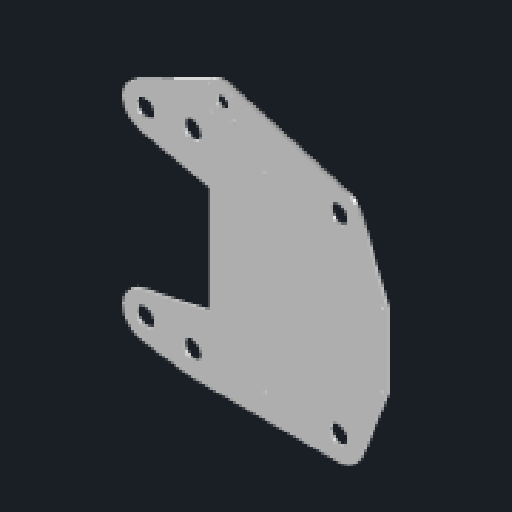
# Autodesk Inventor part: OUTK_002_ShotPlateNoReceptacle
Saved by Autodesk Inventor 2024.2 (Build 282272000, 272)
## iProperties
Created: 2024-11-24
Part Number: OUTK_002_ShotPlateNoReceptacle
Material: Aluminum 6061
Document SubType Name: Modeling
Designer: Bryan
Density: 2.7 g/cm^3
Appearance: Aluminum - Flat
Mass: 844.378 g
Surface Area: 1588.21 cm^2
Volume: 312.733 cm^3
Author: Bryan
Autodesk Inventor part; units mm, degrees
ref_plane "YZ Plane" through (0, 0, 0) normal (1, 0, 0) x (0, 1, 0)
ref_plane "XZ Plane" through (0, 0, 0) normal (0, 1, 0) x (-1, 0, 0)
ref_plane "XY Plane" through (0, 0, 0) normal (0, 0, 1) x (1, 0, 0)
sketch "Sketch1" plane through (0, 0, 0) normal (0, 0, 1) x (1, 0, 0)
  circle A0 centre (239.2032, 0) radius 130.175 projected
  arc A1 (74.585, 187.96) -> (69.5611, 187.6187) centre (74.585, 150.8125) ccw projected
  line L0 (69.5611, 187.6187) -> (-4.7233, 177.4791) projected
  arc A2 (-4.7233, 177.4791) -> (-7.5024, 108.7653) centre (0, 142.875) ccw projected
  line L1 (-7.5024, 108.7653) -> (102.6782, 84.5312) projected
  line L2 (102.6782, 84.5312) -> (102.6782, -84.5312) projected
  line L3 (102.6782, -84.5312) -> (-7.5024, -108.7653) projected
  arc A3 (-7.5024, -108.7653) -> (-5.1627, -177.4163) centre (0, -142.875) ccw projected
  line L4 (-5.1627, -177.4163) -> (68.953, -188.4939) projected
  arc A4 (68.953, -188.4939) -> (74.585, -188.9125) centre (74.585, -150.8125) ccw projected
  line L5 (74.585, -188.9125) -> (305.8782, -188.9125) projected
  arc A5 (305.8782, -188.9125) -> (341.4207, -164.5364) centre (305.8782, -150.8125) ccw projected
  line L6 (341.4207, -164.5364) -> (381.652, -60.3445) projected
  arc A6 (381.652, -60.3445) -> (382.0782, -58.0572) centre (375.7282, -58.0572) ccw projected
  line L7 (382.0782, -58.0572) -> (382.0782, 58.0572) projected
  arc A7 (382.0782, 58.0572) -> (381.6323, 60.3949) centre (375.7282, 58.0572) ccw projected
  line L8 (381.6323, 60.3949) -> (340.4169, 164.488) projected
  arc A8 (340.4169, 164.488) -> (305.8782, 187.96) centre (305.8782, 150.8125) ccw projected
  circle A9 centre (74.585, -150.8125) radius 14.2875 projected
  circle A10 centre (74.585, 150.8125) radius 14.2875 projected
  circle A11 centre (190.2316, 150.8125) radius 3.2512 projected
  circle A12 centre (190.2316, -150.8125) radius 3.2512 projected
  circle A13 centre (375.7282, -58.0572) radius 3.2512 projected
  circle A14 centre (375.7282, 58.0572) radius 3.2512 projected
  circle A15 centre (305.8782, 150.8125) radius 14.2875 projected
  circle A16 centre (305.8782, -150.8125) radius 14.2875 projected
  circle A17 centre (0, -142.875) radius 14.2875 projected
  circle A18 centre (0, 142.875) radius 14.2875 projected
  circle A19 centre (112.9698, 216.6384) radius 38.1 construction
  circle A20 centre (112.9698, 216.6384) radius 19.1008 construction
  circle A21 centre (112.9698, 216.6384) radius 9.6202
  circle A22 centre (133.1724, 201.2431) radius 2.4892
  circle A23 centre (128.3651, 236.841) radius 2.4892
  circle A24 centre (92.7672, 232.0337) radius 2.4892
  circle A25 centre (97.5746, 196.4358) radius 2.4892
  line L9 (84.856, 243.5486) -> (92.7672, 232.0337) construction
  line L10 (128.3651, 236.841) -> (132.9386, 250.0419) construction
  circle A26 centre (112.9698, 216.6384) radius 25.4 construction
  line L11 (112.9698, 216.6384) -> (305.8782, -150.8125) construction
  circle A27 centre (74.585, 150.8125) radius 38.1 construction
  line L12 (318.039, 185.9131) -> (125.4424, 252.639)
  line L13 (91.3948, 248.041) -> (-19.7772, 171.6608)
  arc A28 (125.4424, 252.639) -> (91.3948, 248.041) centre (112.9698, 216.6384) ccw
  dimension "d192" = 50.8
  dimension "d186" = 76.2
  dimension "d187" = 38.2016
  dimension "d188" = 19.2405
  dimension "d189" = 4.9784
  dimension "d190" = 360
  dimension "d193" = 415.0106
  constraints: 10 end point, 9 centre point, 6 coincident, 6 point on circle, 5 tangent, 2 perpendicular, 2 point on line, 1 concentric, 1 equal length, 1 equal radius, 12 other
  measures "d186" diameter of A19
  measures "d187" diameter of A20
  measures "d188" diameter of A21
  measures "d189" diameter of A22
  measures "d193" distance of L11.start L11.end
extrude "Extrusion1" add sketch "Sketch1" along normal mid plane 4.7625 contours A0 | L13 A28 L12 A8 L8 A7 L7 A6 L6 A5 L5 A4 L4 A3 L3 L2 L1 A2
sketch "Sketch2" plane through (0, 0, -2.3813) normal (0, 0, -1) x (-1, 0, 0)
  line L0 (7.573, -108.7809) -> (-101.6, -84.5312) projected
  line L1 (-101.6, -84.5312) -> (-101.6, 84.5312) projected
  line L2 (-101.6, 84.5312) -> (7.573, 108.7809) projected
  arc A0 (7.573, 108.7809) -> (16.0837, 173.8761) centre (0, 142.875) ccw projected
  arc A1 (-315.0883, 186.5069) -> (-339.3386, 164.488) centre (-304.8, 150.8125) ccw projected
  line L3 (-339.3386, 164.488) -> (-380.554, 60.3949) projected
  arc A2 (-380.554, 60.3949) -> (-381, 58.0572) centre (-374.65, 58.0572) ccw projected
  line L4 (-381, 58.0572) -> (-381, -58.0572) projected
  arc A3 (-381, -58.0572) -> (-380.5737, -60.3445) centre (-374.65, -58.0572) ccw projected
  line L5 (-380.5737, -60.3445) -> (-340.3424, -164.5364) projected
  arc A4 (-340.3424, -164.5364) -> (-304.8, -188.9125) centre (-304.8, -150.8125) ccw projected
  line L6 (-304.8, -188.9125) -> (-74.585, -188.9125) projected
  arc A5 (-74.585, -188.9125) -> (-68.953, -188.4939) centre (-74.585, -150.8125) ccw projected
  line L7 (-68.953, -188.4939) -> (5.1627, -177.4163) projected
  arc A6 (5.1627, -177.4163) -> (7.573, -108.7809) centre (0, -142.875) ccw projected
  circle A7 centre (-74.585, -150.8125) radius 14.2875 projected
  circle A8 centre (-74.585, 150.8125) radius 14.2875 projected
  circle A9 centre (-189.6925, 150.8125) radius 3.2512 projected
  circle A10 centre (-189.6925, -150.8125) radius 3.2512 projected
  circle A11 centre (-374.65, -58.0572) radius 3.2512 projected
  circle A12 centre (-374.65, 58.0572) radius 3.2512 projected
  circle A13 centre (-304.8, 150.8125) radius 14.2875 projected
  circle A14 centre (-304.8, -150.8125) radius 14.2875 projected
  circle A15 centre (0, -142.875) radius 14.2875 projected
  circle A16 centre (0, 142.875) radius 14.2875 projected
  line L8 (16.0837, 173.8761) -> (-107.2199, 237.8472) projected
  arc A17 (-107.2199, 237.8472) -> (-129.3442, 240.0442) centre (-121.0355, 211.2177) ccw projected
  line L9 (-129.3442, 240.0442) -> (-315.0883, 186.5069) projected
  line L10 (-101.6, -84.5312) -> (7.573, -108.7809) projected
  arc A18 (5.1627, -177.4163) -> (7.573, -108.7809) centre (0, -142.875) ccw projected
  line L11 (5.1627, -177.4163) -> (-68.953, -188.4939) projected
  arc A19 (-74.585, -188.9125) -> (-68.953, -188.4939) centre (-74.585, -150.8125) ccw projected
  line L12 (-74.585, -188.9125) -> (-304.8, -188.9125) projected
  arc A20 (-340.3424, -164.5364) -> (-304.8, -188.9125) centre (-304.8, -150.8125) ccw projected
  line L13 (-340.3424, -164.5364) -> (-380.5737, -60.3445) projected
  arc A21 (-381, -58.0572) -> (-380.5737, -60.3445) centre (-374.65, -58.0572) ccw projected
  line L14 (-381, -58.0572) -> (-381, 58.0572) projected
  arc A22 (-380.554, 60.3949) -> (-381, 58.0572) centre (-374.65, 58.0572) ccw projected
  line L15 (-380.554, 60.3949) -> (-339.3386, 164.488) projected
  arc A23 (-315.0883, 186.5069) -> (-339.3386, 164.488) centre (-304.8, 150.8125) ccw projected
  line L16 (-315.0883, 186.5069) -> (-129.3442, 240.0442) projected
  arc A24 (-107.2199, 237.8472) -> (-129.3442, 240.0442) centre (-121.0355, 211.2177) ccw projected
  line L17 (-107.2199, 237.8472) -> (16.0837, 173.8761) projected
  arc A25 (7.573, 108.7809) -> (16.0837, 173.8761) centre (0, 142.875) ccw projected
  line L18 (7.573, 108.7809) -> (-101.6, 84.5312) projected
  line L19 (-101.6, 84.5312) -> (-101.6, -84.5312) projected
  circle A26 centre (-74.585, -150.8125) radius 14.2875 projected
  circle A27 centre (-74.585, 150.8125) radius 14.2875 projected
  circle A28 centre (-189.6925, 150.8125) radius 3.2512 projected
  circle A29 centre (-189.6925, -150.8125) radius 3.2512 projected
  circle A30 centre (-374.65, -58.0572) radius 3.2512 projected
  circle A31 centre (-374.65, 58.0572) radius 3.2512 projected
  circle A32 centre (-304.8, 150.8125) radius 14.2875 projected
  circle A33 centre (-304.8, -150.8125) radius 14.2875 projected
  circle A34 centre (0, -142.875) radius 14.2875 projected
  circle A35 centre (0, 142.875) radius 14.2875 projected
  circle A36 centre (-121.0355, 211.2177) radius 9.6202 projected
  circle A37 centre (-140.6829, 195.1199) radius 2.4892 projected
  circle A38 centre (-137.1333, 230.8651) radius 2.4892 projected
  circle A39 centre (-101.3881, 227.3155) radius 2.4892 projected
  circle A40 centre (-104.9377, 191.5703) radius 2.4892 projected
  line L20 (0, 142.875) -> (-74.585, 150.8125)
  line L21 (-74.585, 150.8125) -> (-121.0355, 211.2177)
  line L22 (-121.0355, 211.2177) -> (-189.6925, 150.8125)
  line L23 (-189.6925, 150.8125) -> (-304.8, 150.8125)
  line L24 (-304.8, 150.8125) -> (-374.65, 58.0572)
  line L25 (-374.65, 58.0572) -> (-374.65, -58.0572)
  line L26 (-374.65, -58.0572) -> (-304.8, -150.8125)
  line L27 (-304.8, -150.8125) -> (-189.6925, -150.8125)
  line L28 (-189.6925, -150.8125) -> (-74.585, -150.8125)
  line L29 (-74.585, -150.8125) -> (0, -142.875)
  line L30 (-0.504, -138.1392) -> (-74.8377, -146.05)
  line L31 (-74.8377, -146.05) -> (-189.6925, -146.05)
  line L32 (-189.6925, -146.05) -> (-302.4246, -146.05)
  line L33 (-302.4246, -146.05) -> (-369.8875, -56.4646)
  line L34 (-369.8875, -56.4646) -> (-369.8875, 56.4646)
  line L35 (-369.8875, 56.4646) -> (-302.4246, 146.05)
  line L36 (-302.4246, 146.05) -> (-187.8957, 146.05)
  line L37 (-187.8957, 146.05) -> (-121.7094, 204.2814)
  line L38 (-121.7094, 204.2814) -> (-77.1171, 146.2926)
  line L39 (-77.1171, 146.2926) -> (-0.504, 138.1392)
  circle A41 centre (-121.0355, 211.2177) radius 30
  line L40 (-121.0355, 211.2177) -> (0, 142.875)
  line L41 (-304.8, 150.8125) -> (-121.0355, 211.2177)
  line L42 (-121.546, 206.0367) -> (-22.3877, 150.0469)
  line L43 (-22.3877, 150.0469) -> (-72.053, 155.3324)
  line L44 (-72.053, 155.3324) -> (-120.3616, 218.154)
  line L45 (-120.3616, 218.154) -> (-191.4893, 155.575)
  line L46 (-191.4893, 155.575) -> (-275.0604, 155.575)
  line L47 (-275.0604, 155.575) -> (-121.546, 206.0367)
  line L48 (-374.65, 58.0572) -> (-247.2463, 0)
  line L49 (-374.65, -58.0572) -> (-247.2463, 0)
  line L50 (-377.9363, 54.3211) -> (-258.7313, 0)
  line L51 (-258.7313, 0) -> (-381.225, -55.8197)
  line L52 (-371.4001, 61.81) -> (-235.7612, 0)
  line L53 (-235.7612, 0) -> (-375.2, -63.5416)
  line L54 (-189.6925, 150.8125) -> (-247.2463, 0)
  line L55 (-247.2463, 0) -> (-189.6925, -150.8125)
  line L56 (-74.585, 150.8125) -> (-189.6925, 150.8125)
  line L57 (-74.585, 150.8125) -> (-101.6, 84.5312)
  line L58 (-74.585, -150.8125) -> (-101.6, -84.5312)
  line L59 (-187.5785, 142.9947) -> (-252.4177, -26.9086)
  line L60 (-195.5097, 148.9267) -> (-260.349, -20.9767)
  line L61 (-256.7203, 11.4682) -> (-192.2893, -157.3653)
  line L62 (-248.8555, 17.5743) -> (-184.4245, -151.2592)
  line L63 (-78.9953, -152.61) -> (-106.0102, -86.3287)
  line L64 (-70.1748, -149.015) -> (-97.1898, -82.7337)
  line L65 (-78.9953, 152.61) -> (-106.0102, 86.3287)
  line L66 (-106.3625, 88.3519) -> (-106.3625, -88.3519)
  line L67 (-106.3625, -88.3519) -> (6.5404, -113.4301)
  arc A42 (4.4587, -172.7061) -> (6.5404, -113.4301) centre (0, -142.875) ccw
  line L68 (4.4587, -172.7061) -> (-69.657, -183.7838)
  arc A43 (-74.585, -184.15) -> (-69.657, -183.7838) centre (-74.585, -150.8125) ccw
  line L69 (-74.585, -184.15) -> (-304.8, -184.15)
  arc A44 (-335.8996, -162.8209) -> (-304.8, -184.15) centre (-304.8, -150.8125) ccw
  line L70 (-335.8996, -162.8209) -> (-376.1309, -58.6291)
  arc A45 (-376.2375, -58.0572) -> (-376.1309, -58.6291) centre (-374.65, -58.0572) ccw
  line L71 (-376.2375, -58.0572) -> (-376.2375, 58.0572)
  arc A46 (-376.126, 58.6416) -> (-376.2375, 58.0572) centre (-374.65, 58.0572) ccw
  line L72 (-376.126, 58.6416) -> (-334.9106, 162.7347)
  arc A47 (-313.7692, 181.9307) -> (-334.9106, 162.7347) centre (-304.8, 150.8125) ccw
  line L73 (-313.7692, 181.9307) -> (-128.0252, 235.468)
  arc A48 (-109.4131, 233.6198) -> (-128.0252, 235.468) centre (-121.0355, 211.2177) ccw
  line L74 (-109.4131, 233.6198) -> (13.8905, 169.6487)
  arc A49 (6.5404, 113.4301) -> (13.8905, 169.6487) centre (0, 142.875) ccw
  line L75 (6.5404, 113.4301) -> (-106.3625, 88.3519)
  line L76 (-247.2463, 0) -> (-106.3625, 0)
  line L77 (-189.6925, 150.8125) -> (-106.3625, 0)
  line L78 (-106.3625, 0) -> (-189.6925, -150.8125)
  line L79 (-193.861, 148.5092) -> (-110.531, -2.3033)
  line L80 (-185.524, 153.1158) -> (-102.194, 2.3033)
  line L81 (-305.5222, -4.7625) -> (-107.2014, -4.7625)
  line L82 (-305.8488, 4.7625) -> (-107.528, 4.7625)
  line L83 (-110.531, 2.3033) -> (-193.861, -148.5092)
  line L84 (-102.194, -2.3033) -> (-185.524, -153.1158)
  line L85 (-74.585, 146.05) -> (-189.6925, 146.05)
  line L86 (-74.585, 155.575) -> (-189.6925, 155.575)
  line L87 (-101.6, 84.5312) -> (-148.0275, 75.4063)
  line L88 (-101.6, -84.5312) -> (-148.0275, -75.4062)
  line L89 (-148.946, 80.0793) -> (-105.0402, 88.7087)
  line L90 (-105.0402, 88.7087) -> (-78.9953, 152.61)
  line L91 (-147.109, 70.7332) -> (-98.1598, 80.3537)
  line L92 (-98.1598, 80.3537) -> (-70.1748, 149.015)
  line L93 (-148.946, -80.0793) -> (-105.0402, -88.7087)
  line L94 (-105.0402, -88.7087) -> (-78.9953, -152.61)
  line L95 (-147.109, -70.7332) -> (-98.1598, -80.3537)
  line L96 (-98.1598, -80.3537) -> (-70.1748, -149.015)
  circle A50 centre (-74.585, -150.8125) radius 19.05
  circle A51 centre (-304.8, -150.8125) radius 19.05
  circle A52 centre (-304.8, 150.8125) radius 19.05
  circle A53 centre (-189.6925, 150.8125) radius 8.0137
  circle A54 centre (-189.6925, -150.8125) radius 8.0137
  circle A55 centre (-74.585, 150.8125) radius 19.05
  circle A56 centre (-374.65, 58.0572) radius 6.35
  line L97 (-101.6, 84.5312) -> (-101.6, -84.5312) projected
  line L98 (-304.8, 150.8125) -> (-247.2463, 0)
  line L99 (-304.8, -150.8125) -> (-247.2463, 0)
  line L100 (-309.2495, 149.1145) -> (-251.6958, -1.698)
  line L101 (-300.3505, 152.5105) -> (-242.7968, 1.698)
  line L102 (-300.3505, -152.5105) -> (-242.7968, -1.698)
  line L103 (-309.2495, -149.1145) -> (-251.6958, 1.698)
  point P0 (-93.0301, -146.05)
  point P1 (-85.9571, -135.5292)
  point P2 (-145.5385, -80.7491)
  point P3 (-181.6199, -146.05)
  point P4 (-140.7003, -71.9927)
  point P5 (-106.3625, -78.7416)
  point P6 (-106.3625, -9.8475)
  point P7 (-286.3549, -146.05)
  point P8 (-196.6075, -146.05)
  point P9 (-312.0914, -133.2131)
  point P10 (-367.277, -59.9311)
  point P11 (-369.8875, -50.6533)
  point P12 (-369.8875, 50.6533)
  point P13 (-312.0914, 133.2131)
  point P14 (-367.277, 59.9311)
  point P15 (-188.9002, -139.5311)
  point P16 (-114.4351, -4.7625)
  point P17 (-240.3313, -4.7625)
  point P18 (-240.3313, 4.7625)
  point P19 (-114.4351, 4.7625)
  point P20 (-188.9002, 139.5311)
  point P21 (-106.3625, 78.7416)
  point P22 (-140.7003, 71.9927)
  point P23 (-106.3625, 9.8475)
  point P24 (-286.3549, 146.05)
  point P25 (-196.6075, 146.05)
  point P26 (-196.1375, 155.575)
  point P27 (-187.9996, 158.6453)
  point P28 (-146.4193, 195.2282)
  point P29 (-147.6867, 197.444)
  point P30 (-85.9571, 135.5292)
  point P31 (-93.0301, 146.05)
  point P32 (-181.6199, 146.05)
  point P33 (-145.5385, 80.7491)
  point P34 (-93.0301, 155.575)
  point P35 (-89.6042, 162.5311)
  point P36 (-106.7552, 184.8346)
  point P37 (-140.1275, 188.077)
  point P38 (-177.0695, 155.575)
  point P39 (-82.0536, 168.3374)
  point P40 (-55.7395, 153.5963)
  point P41 (-97.5852, 192.5072)
  point P42 (-99.2045, 190.6409)
  point P43 (-247.2463, 150.8125)
  point P44 (-101.6, 0)
  point P45 (-302.673, -131.8816)
  point P46 (-260.349, -20.9767)
  point P47 (-255.8346, -9.1474)
  point P48 (-252.4177, -26.9086)
  point P49 (-293.774, -135.2777)
  point P50 (-247.2463, -13.3574)
  point P51 (-293.774, 135.2777)
  point P52 (-247.2463, 13.3574)
  point P53 (-302.673, 131.8816)
  point P54 (-255.8346, 9.1474)
  point P55 (-369.8875, 53.8571)
  point P56 (-368.319, 58.5475)
  dimension "d123" = 4.7625
  dimension "d124" = 60
  dimension "d125" = 4.7625
  dimension "d126" = 4.7625
  dimension "d127" = 4.7625
  dimension "d130" = 4.7625
  dimension "d131" = 4.7625
  dimension "d132" = 4.7625
  dimension "d133" = 4.7625
  dimension "d134" = 4.7625
  dimension "d135" = 4.7625
  dimension "d136" = 4.7625
  dimension "d137" = 4.7625
  dimension "d138" = 4.7625
  dimension "d139" = 4.7625
  dimension "d140" = 4.7625
  dimension "d141" = 4.7625
  dimension "d142" = 4.7625
  dimension "d143" = 4.7625
  dimension "d144" = 4.7625
  dimension "d145" = 4.7625
  dimension "d146" = 4.7625
  dimension "d147" = 4.7625
  dimension "d148" = 4.7625
  dimension "d149" = 4.7625
  dimension "d150" = 4.7625
  dimension "d151" = 4.7625
  dimension "d152" = 4.7625
  dimension "d153" = 4.7625
  dimension "d154" = 4.7625
  dimension "d155" = 4.7625
  dimension "d157" = 12.7
  dimension "d158" = 4.7625
  dimension "d159" = 4.7625
  dimension "d160" = 4.7625
  dimension "d161" = 4.7625
  constraints: 166 end point, 19 parallel, 16 centre point, 16 point on circle, 5 midpoint, 4 horizontal, 2 coincident, 1 horizontal alignment, 1 vertical, 1 vertical alignment, 37 other
  measures "d123" distance between parallel lines of L23 L36
  measures "d124" diameter of A41
  measures "d125" distance between parallel lines of L41 L47
  measures "d126" distance between parallel lines of L48 L50
  measures "d127" distance between parallel lines of L48 L52
  measures "d130" distance between parallel lines of L54 L59
  measures "d131" distance between parallel lines of L54 L60
  measures "d132" distance between parallel lines of L55 L61
  measures "d133" distance between parallel lines of L55 L62
  measures "d134" distance between parallel lines of L58 L63
  measures "d135" distance between parallel lines of L58 L64
  measures "d136" distance between parallel lines of L57 L65
  measures "d137" distance between parallel lines of L1 L66
  measures "d138" distance between parallel lines of L77 L79
  measures "d139" distance between parallel lines of L77 L80
  measures "d140" distance between parallel lines of L76 L81
  measures "d141" distance between parallel lines of L76 L82
  measures "d142" distance between parallel lines of L78 L83
  measures "d143" distance between parallel lines of L78 L84
  measures "d144" distance between parallel lines of L56 L85
  measures "d145" distance between parallel lines of L56 L86
  measures "d146" distance between parallel lines of L87 L89
  measures "d147" distance between parallel lines of L87 L91
  measures "d148" distance between parallel lines of L88 L93
  measures "d149" distance between parallel lines of L88 L95
  measures "d150" radial gap between concentric circles of A7 A50
  measures "d151" radial gap between concentric circles of A14 A51
  measures "d152" radial gap between concentric circles of A13 A52
  measures "d153" radial gap between concentric circles of A9 A53
  measures "d154" radial gap between concentric circles of A10 A54
  measures "d155" radial gap between concentric circles of A8 A55
  measures "d157" diameter of A56
  measures "d158" distance between parallel lines of L98 L100
  measures "d159" distance between parallel lines of L98 L101
  measures "d160" distance between parallel lines of L99 L102
  measures "d161" distance between parallel lines of L99 L103
extrude "Not Final Pocketing" [suppressed]
fillet "Fillet3" [suppressed]
sketch "Sketch3" plane through (0, 0, 2.3813) normal (0, 0, 1) x (1, 0, 0)
  circle A0 centre (248.2641, 7.8919) radius 3.2512
  circle A1 centre (252.7796, -17.1035) radius 3.2512
  line L0 (248.2641, 7.8919) -> (248.2641, -17.1035)
  line L1 (248.2641, -17.1035) -> (252.7796, -17.1035)
  line L2 (252.7796, -17.1035) -> (248.2641, 7.8919)
  arc A2 (241.3136, 28.9032) -> (253.1789, 28.9032) centre (247.2463, 31.1673) ccw projected
  line L3 (247.5237, 24.8234) -> (248.2641, 7.8919)
  arc A3 (261.3531, 23.6079) -> (269.9189, 15.5655) centre (267.2858, 21.3438) ccw projected
  line L4 (262.1012, 17.6774) -> (248.2641, 7.8919)
  arc A4 (253.1789, -28.9032) -> (241.3136, -28.9032) centre (247.2463, -31.1673) ccw projected
  line L5 (249.5712, -25.2582) -> (252.7796, -17.1035)
  line L6 (252.7796, -17.1035) -> (261.1908, -19.5622)
  arc A5 (269.9189, -15.5655) -> (261.3531, -23.6079) centre (267.2858, -21.3438) ccw projected
  point P0 (0, 0)
  dimension "d162" = 6.5024
  dimension "d163" = 25.4
  dimension "d164" = 10.24
  constraints: 14 end point, 4 point on circle, 4 point on line, 2 centre point, 2 equal length, 1 equal radius, 1 perpendicular, 1 vertical
  measures "d162" diameter of A0
  measures "d163" distance of L1.end L0.start
  measures "d164" angle of L2 L0
hole "Hole1" [suppressed]
sketch "Sketch4" plane through (0, 0, 2.3813) normal (0, 0, 1) x (1, 0, 0)
  circle A0 centre (248.2641, 7.8919) radius 3.2512 projected
  circle A1 centre (252.7796, -17.1035) radius 3.2512 projected
  line L0 (248.2641, 7.8919) -> (252.7796, -17.1035)
  line L1 (248.2641, 7.8919) -> (212.1396, 207.8551)
  circle A2 centre (212.1396, 207.8551) radius 3.8059
  circle A3 centre (216.6552, 182.8597) radius 8.1342
  point P0 (0, 0)
  dimension "d172" = 203.2
  dimension "d173" = 25.4
  constraints: 4 end point, 2 centre point, 1 coincident, 1 collinear, 1 point on line
  measures "d172" distance of L0.start L1.end
  measures "d173" distance of A3.centre L1.end
hole "Hole2" [suppressed]
sketch "Sketch5" plane through (0, 0, 2.3813) normal (0, 0, 1) x (1, 0, 0)
  arc A0 (340.4169, 164.488) -> (318.039, 185.9131) centre (305.8782, 150.8125) ccw projected
  arc A1 (381.652, -60.3445) -> (382.0782, -58.0572) centre (375.7282, -58.0572) ccw projected
  line L0 (74.585, -188.9125) -> (305.8782, -188.9125) projected
  arc A2 (125.4424, 252.639) -> (91.3948, 248.041) centre (112.9698, 216.6384) ccw projected
  circle A3 centre (375.7282, -58.0572) radius 3.2512 projected
  circle A4 centre (375.7282, 58.0572) radius 3.2512 projected
  circle A5 centre (305.8782, 150.8125) radius 14.2875 projected
  circle A6 centre (305.8782, -150.8125) radius 14.2875 projected
  circle A7 centre (0, -142.875) radius 14.2875 projected
  circle A8 centre (0, 142.875) radius 14.2875 projected
  circle A9 centre (92.7672, 232.0337) radius 2.4892 projected
  circle A10 centre (133.1724, 201.2431) radius 2.4892 projected
  circle A11 centre (128.3651, 236.841) radius 2.4892 projected
  circle A12 centre (74.585, -150.8125) radius 14.2875 projected
  circle A13 centre (74.585, 150.8125) radius 14.2875 projected
  circle A14 centre (190.2316, 150.8125) radius 3.2512 projected
  circle A15 centre (190.2316, -150.8125) radius 3.2512 projected
  circle A16 centre (112.9698, 216.6384) radius 9.6202 projected
  circle A17 centre (97.5746, 196.4358) radius 2.4892 projected
  line L1 (-7.5024, 108.7653) -> (102.6782, 84.5312) projected
  line L2 (102.6782, 84.5312) -> (102.6782, -84.5312) projected
  line L3 (102.6782, -84.5312) -> (-7.5024, -108.7653) projected
  arc A18 (-7.5024, -108.7653) -> (-5.1627, -177.4163) centre (0, -142.875) ccw projected
  line L4 (-5.1627, -177.4163) -> (68.953, -188.4939) projected
  arc A19 (68.953, -188.4939) -> (74.585, -188.9125) centre (74.585, -150.8125) ccw projected
  line L5 (74.585, -188.9125) -> (305.8782, -188.9125) projected
  arc A20 (305.8782, -188.9125) -> (341.4207, -164.5364) centre (305.8782, -150.8125) ccw projected
  line L6 (341.4207, -164.5364) -> (381.652, -60.3445) projected
  arc A21 (381.652, -60.3445) -> (382.0782, -58.0572) centre (375.7282, -58.0572) ccw projected
  line L7 (382.0782, -58.0572) -> (382.0782, 58.0572) projected
  arc A22 (382.0782, 58.0572) -> (381.6323, 60.3949) centre (375.7282, 58.0572) ccw projected
  line L8 (381.6323, 60.3949) -> (340.4169, 164.488) projected
  arc A23 (340.4169, 164.488) -> (318.039, 185.9131) centre (305.8782, 150.8125) ccw projected
  line L9 (318.039, 185.9131) -> (125.4424, 252.639) projected
  arc A24 (125.4424, 252.639) -> (91.3948, 248.041) centre (112.9698, 216.6384) ccw projected
  line L10 (91.3948, 248.041) -> (-19.7772, 171.6608) projected
  arc A25 (-19.7772, 171.6608) -> (-7.5024, 108.7653) centre (0, 142.875) ccw projected
  line L11 (107.8709, 254.3956) -> (308.2734, 281.4591)
  line L12 (308.2734, 281.4591) -> (341.6806, 160.7185)
  point P0 (0, 0)
  point P1 (381.9708, -59.2206)
  point P2 (318.039, 185.9131)
  point P3 (340.4169, 164.488)
  point P4 (381.652, -60.3445)
  point P5 (341.1497, 162.6371)
  dimension "d202" = 74.534
  constraints: 4 end point, 3 point on circle, 2 tangent
  measures "d202" angle of L0 L12
extrude "Extrusion3" add sketch "Sketch5" against normal up to surface (4.7625 mm away) contours A0 L9 A2 L11 L12 L8
sketch "Sketch7" plane through (0, 0, 2.3813) normal (0, 0, 1) x (1, 0, 0)
  circle A0 centre (299.4199, 265.8323) radius 3.4686
  line L0 (299.4199, 265.8323) -> (306.1933, 241.3521)
  line L1 (306.1933, 241.3521) -> (312.9666, 216.8718)
  line L2 (341.1497, 162.6371) -> (308.2734, 281.4591) projected
  line L3 (308.2734, 281.4591) -> (256.5939, 267.1601)
  line L4 (312.9666, 216.8718) -> (350.617, 80.7953)
  line L5 (350.617, 80.7953) -> (375.7282, -9.9618)
  circle A1 centre (375.7282, 58.0572) radius 3.2512 projected
  point P0 (0, 0)
  dimension "d203" = 25.4
  dimension "d204" = 25.4
  dimension "d205" = 12.7
  dimension "d206" = 12.7
  dimension "d207" = 235.3562
  constraints: 10 end point, 2 point on line, 1 centre point, 1 collinear, 1 parallel, 1 perpendicular, 1 vertical alignment
  measures "d203" distance of L0.start L0.end
  measures "d204" distance of L0.end L1.end
  measures "d205" distance between parallel lines of L2 L0
  measures "d206" distance from line of L0.start L3
  measures "d207" distance of L5.end L1.end
hole "Hole3" at (299.4199, 265.8323, 2.3813) at (306.1933, 241.3521, 2.3813) at (312.9666, 216.8718, 2.3813) at (375.7282, -9.9618, 2.3813) direction (0, 0, -1) diameter 6.5024 depth 4.7625 tip angle 118
fillet "Fillet4" radius 12.7 1 edges at (308.2734, 281.4591, 0)
body "Solid1"
